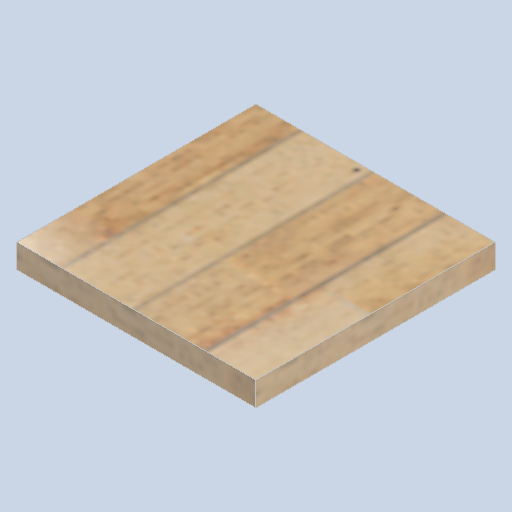
# Autodesk Inventor part: Part3
Saved by Autodesk Inventor 2022 (Build 260153000, 153)
## iProperties
Created: 2022-04-11
Part Number: Part3
Material: Wood (Maple)
Document SubType Name: Modeling
Designer: MacBook
Density: 0.67 g/cm^3
Appearance: Natural Maple - Glossy Dark Tint
Author: MacBook
Autodesk Inventor part; units mm, degrees
ref_plane "YZ Plane" through (0, 0, 0) normal (1, 0, 0) x (0, 1, 0)
ref_plane "XZ Plane" through (0, 0, 0) normal (0, 1, 0) x (-1, 0, 0)
ref_plane "XY Plane" through (0, 0, 0) normal (0, 0, 1) x (1, 0, 0)
sketch "Sketch1" plane through (0, 0, 0) normal (0, 1, 0) x (-1, 0, 0)
  line L0 (-94.4563, -94.4563) -> (94.4562, -94.4563)
  line L1 (94.4562, -94.4563) -> (94.4562, 94.4562)
  line L2 (94.4562, 94.4562) -> (-94.4562, 94.4562)
  line L3 (-94.4562, 94.4562) -> (-94.4563, -94.4563)
  line L4 (-94.4563, -94.4563) -> (94.4562, 94.4562) construction
  line L5 (94.4562, -94.4563) -> (-94.4562, 94.4562) construction
  point P0 (0, 0)
  dimension "d0" = 188.9125
  dimension "d1" = 188.9125
  constraints: 12 end point, 2 midpoint, 2 parallel, 1 horizontal, 1 perpendicular
  measures "d0" distance between parallel lines of L3 L1
  measures "d1" distance between parallel lines of L0 L2
extrude "Extrusion1" add sketch "Sketch1" against normal blind 19.05
body "Solid1"
